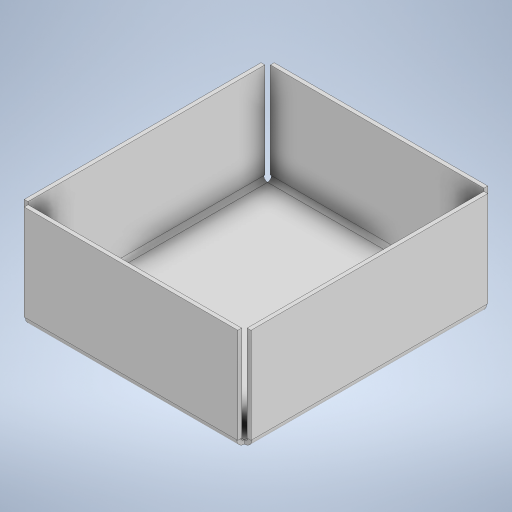
# Autodesk Inventor part: Part37
Saved by Autodesk Inventor 2024.3 (Build 283343000, 343)
## iProperties
Created: 2025-06-19
Part Number: Part37
Material: Generic
Document SubType Name: Sheet Metal
Designer: ajclo
Density: 1 g/cm^3
Sheet Metal Rule: Default_mm
Appearance: Default
Flat Pattern Width: 16.2786 cm
Flat Pattern Length: 17.1786 cm
Flat Pattern Area: 279.643 cm^2
Sheet Metal Width: 162,786 mm
Sheet Metal Length: 171,786 mm
Sheet Metal Area: 27964,302 mm^2
Author: ajclo
Autodesk Inventor part; units mm, degrees
note: some values were not read from the file. Chosen so that the rebuilt part matches the saved one: corner form of "Plate2".
ref_plane "YZ Plane" through (0, 0, 0) normal (1, 0, 0) x (0, 1, 0)
ref_plane "XZ Plane" through (0, 0, 0) normal (0, 1, 0) x (-1, 0, 0)
ref_plane "XY Plane" through (0, 0, 0) normal (0, 0, 1) x (1, 0, 0)
sketch "Sketch1" plane through (0, 0, 0) normal (0, 1, 0) x (-1, 0, 0)
  line L0 (0, 0) -> (88, 0)
  line L1 (88, 0) -> (88, -97)
  line L2 (88, -97) -> (0, -97)
  line L3 (0, -97) -> (0, 0)
  dimension "d0" = 97
  dimension "d1" = 88
  measures "d0" distance of L0.end L1.end
  measures "d1" distance of L1.end L2.end
extrude "Plate1" add sketch "Sketch1" along normal blind 1.5
sketch "Sketch2" plane through (-86.5, 0, 0) normal (-1, 0, 0) x (0, -1, 0)
  line L0 (0, -97) -> (0, 0)
  line L1 (0, 0) -> (-40, 0)
  line L2 (-40, 0) -> (-40, -97)
  line L3 (-40, -97) -> (0, -97)
  constraints: 6 end point, 1 horizontal, 1 perpendicular, 1 vertical
edge flange "Flange1" height 40 angle 90 thickness 1.5 bend radius 1.5 thickness toward (-1, 0, 0) relief tear relief width 1.5 relief depth 0.75 corner gap 1.5 corner form 2 edges at (-88, 1.5, -48.5) (-44, 1.5, 0) (0, 1.5, -48.5) (-44, 1.5, -97) wall of the first edge with corners at (-86.5, 0, -97) (-86.5, 0, 0) (-86.5, 40, 0) (-86.5, 40, -97)
bend "Bend1"
corner "Corner1"
equation "\"d2\" = Thickness"
equation "\"d3\" = BendReliefWidth"
equation "\"d4\" = BendReliefDepth"
equation "\"d5\" = MinimumRemnant"
equation "\"d6\" = TransitionRadius"
equation "\"d9\" = BendRadius"
equation "\"d10\" = CornerReliefSize"
equation "\"d11\" = GapSize"
equation "\"d12\" = JacobiRadiusSize"
equation "\"BendRadius\" = Thickness"
equation "\"BendReliefWidth\" = Thickness"
equation "\"BendReliefDepth\" = 0.5 * Thickness"
equation "\"CornerReliefSize\" = 4 * Thickness"
equation "\"MinimumRemnant\" = 2 * Thickness"
equation "\"TransitionRadius\" = BendRadius"
equation "\"JacobiRadiusSize\" = BendRadius"
equation "\"GapSize\" = Thickness"
equation "\"Thickness\" = 1.5"
body "Solid1"
